# Autodesk Inventor part: DX3D-SF
Saved by Autodesk Inventor 2013 (Build 170138000, 138)
## iProperties
Created: 2013-01-27
Part Number: DX3D-SF
Material: Generic
Document SubType Name: Modeling
Designer: davidgitz
Density: 1 g/cm^3
Author: davidgitz
Autodesk Inventor part; units mm, degrees
ref_plane "YZ Plane" through (0, 0, 0) normal (1, 0, 0) x (0, 1, 0)
ref_plane "XZ Plane" through (0, 0, 0) normal (0, 1, 0) x (-1, 0, 0)
ref_plane "XY Plane" through (0, 0, 0) normal (0, 0, 1) x (1, 0, 0)
sketch "DM3D-SF, DX3D-SF_53" plane through (0, 0, 0) normal (0, 0, 1) x (1, 0, 0)
  line L0 (-5.8928, 9.271) -> (7.0612, 9.271)
  line L1 (7.0612, 9.271) -> (7.0612, -3.0988)
  line L2 (7.0612, -3.0988) -> (5.9944, -3.0988)
  line L3 (5.9944, -3.0988) -> (5.6642, -2.794)
  line L4 (5.6642, -2.794) -> (5.6642, -1.1938)
  line L5 (5.6642, -1.1938) -> (-4.4958, -1.1938)
  line L6 (-4.4958, -1.1938) -> (-4.4958, -2.794)
  line L7 (-4.4958, -2.794) -> (-4.8006, -3.0988)
  line L8 (-4.8006, -3.0988) -> (-5.8928, -3.0988)
  line L9 (-5.8928, -3.0988) -> (-5.8928, 9.271)
  constraints: 20 end point
extrude "Extrusion1" add sketch "DM3D-SF, DX3D-SF_53" along normal blind 6.35
body "Solid1"
